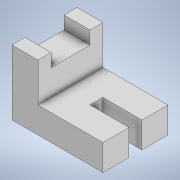
# Autodesk Inventor part: 10-18-19 A
Saved by Autodesk Inventor 2020 (Build 240168000, 168)
## iProperties
Created: 2019-10-18
Part Number: 10-18-19 A
Material: Generic
Document SubType Name: Modeling
Designer: cks4a449
Density: 1 g/cm^3
Appearance: Default
Author: cks4a449
Autodesk Inventor part; units mm, degrees
ref_plane "YZ Plane" through (0, 0, 0) normal (1, 0, 0) x (0, 1, 0)
ref_plane "XZ Plane" through (0, 0, 0) normal (0, 1, 0) x (-1, 0, 0)
ref_plane "XY Plane" through (0, 0, 0) normal (0, 0, 1) x (1, 0, 0)
sketch "Sketch1" plane through (0, 0, 0) normal (0, 0, 1) x (1, 0, 0)
  line L0 (0, 0) -> (9.2453, 0)
  line L1 (0, 0) -> (177.8, 0)
  line L2 (177.8, 0) -> (177.8, 50.8)
  line L3 (177.8, 50.8) -> (50.8, 50.8)
  line L4 (50.8, 50.8) -> (50.8, 127)
  line L5 (50.8, 127) -> (0, 127)
  line L6 (0, 127) -> (0, 0)
  dimension "d0" = 177.8
  dimension "d1" = 50.8
  dimension "d2" = 127
  dimension "d3" = 76.2
  dimension "d4" = 50.8
  constraints: 14 end point, 3 perpendicular, 2 horizontal, 1 point on line
  measures "d0" distance of L0.start L1.end
  measures "d1" distance of L1.end L2.end
  measures "d2" distance of L2.end L3.end
  measures "d3" distance of L3.end L4.end
  measures "d4" distance of L4.end L5.end
extrude "Extrusion1" add sketch "Sketch1" along normal blind 127
sketch "Sketch2" plane through (177.8, 0, 0) normal (1, 0, 0) x (0, 0, -1)
  line L0 (0, 50.8) -> (-127, 50.8) projected
  line L1 (-63.5, 50.8) -> (-50.8, 50.8)
  line L2 (-50.8, 50.8) -> (-76.2, 50.8)
  line L3 (-76.2, 50.8) -> (-76.2, 0)
  line L4 (-76.2, 0) -> (-50.8, 0)
  line L5 (-50.8, 0) -> (-50.8, 50.8)
  point P0 (0, 0)
  dimension "d7" = 12.7
  dimension "d8" = 25.4
  dimension "d9" = 50.8
  constraints: 10 end point, 2 parallel, 1 horizontal, 1 midpoint, 1 perpendicular, 1 point on line
  measures "d7" distance of L1.start L1.end
  measures "d8" distance of L4.end L3.end
  measures "d9" distance of L3.end L2.end
extrude "Extrusion2" cut sketch "Sketch2" against normal blind 76.2
sketch "Sketch3" plane through (0, 127, 0) normal (0, 1, 0) x (1, 0, 0)
  line L0 (0, 0) -> (0, -127) projected
  line L1 (0, -63.5) -> (0, -101.6)
  line L2 (0, -101.6) -> (50.8, -101.6)
  line L3 (50.8, -101.6) -> (50.8, -25.4)
  line L4 (50.8, -25.4) -> (0, -25.4)
  line L5 (0, -25.4) -> (0, -101.6)
  dimension "d12" = 38.1
  dimension "d13" = 50.8
  dimension "d14" = 76.2
  constraints: 10 end point, 2 parallel, 1 horizontal, 1 midpoint, 1 perpendicular, 1 point on line
  measures "d12" distance of L1.start L1.end
  measures "d13" distance of L4.end L3.end
  measures "d14" distance of L3.end L2.end
extrude "Extrusion3" cut sketch "Sketch3" against normal blind 25.4
body "Solid1"
